part2_v6 (Autodesk Fusion 360 design; units mm, degrees)
Autodesk Fusion 360 part; units mm, degrees
sketch "Sketch1" plane through (0, 0, 0) normal (0, 1, 0) x (1, 0, 0)
  line L0 (5.0799, 0.3129) -> (55.0799, 0.3129)
  line L1 (55.0799, 0.3129) -> (55.0799, -174.6871)
  line L2 (55.0799, -174.6871) -> (5.0799, -174.6871)
  line L3 (5.0799, -174.6871) -> (5.0799, 0.3129)
  line L4 (30.0799, 0.3129) -> (30.0799, -174.6871) construction
  line L5 (5.0799, -94.6871) -> (55.0799, -94.6871)
  line L6 (55.0799, -94.6871) -> (55.0799, -79.6871)
  line L7 (55.0799, -79.6871) -> (5.0799, -79.6871)
  line L8 (5.0799, -79.6871) -> (5.0799, -94.6871)
  line L9 (5.0799, -94.6871) -> (55.0799, -79.6871) construction
  line L10 (55.0799, -94.6871) -> (5.0799, -79.6871) construction
  point P0 (30.0799, -87.1871)
  dimension "d2" = 175
  dimension "d11" = 50
  dimension "d12" = 15
  dimension "d37" = 50
  constraint horizontal L0
  constraint vertical L1
  constraint horizontal L2
  constraint midpoint L0 L4.start
  constraint midpoint L2 L4.end
  constraint horizontal L5
  constraint perpendicular L5 L6
  constraint parallel L5 L7
  constraint parallel L6 L8
  constraint coincident L9 P0
  constraint coincident L10 P0
  constraint midpoint L4 P0
  constraint vertical L3
  measures "d2" distance of L0.start L2.end
  measures "d11" distance of L6.end L7.end
  measures "d12" distance of L5.end L6.end
  measures "d37" distance of L0.start L0.end
extrude "Extrude1" add sketch "Sketch1" against normal blind 5
extrude "Extrude3" add sketch "Sketch1" along normal blind 45 contours L1 L3 L5 L6 L7 L8
sketch "Sketch2" plane through (0, 0, 94.6871) normal (0, 0, 1) x (1, 0, 0)
  line L0 (5.0799, 0) -> (55.0799, 0)
  line L1 (55.0799, 0) -> (55.0799, 45)
  line L2 (55.0799, 45) -> (5.0799, 45)
  line L3 (5.0799, 45) -> (5.0799, 0)
  circle A0 centre (30, 27.5) radius 5.35
  line L4 (55.0799, -5) -> (5.0799, -5)
  circle A1 centre (30, 27.5) radius 8
  line L5 (38, 27.5) -> (22, 27.5) construction
  line L6 (30, 19.5) -> (30, 35.5) construction
  circle A2 centre (22, 27.5) radius 2.05
  circle A3 centre (30, 19.5) radius 2.05
  circle A4 centre (38, 27.5) radius 2.05
  circle A5 centre (30, 35.5) radius 2.05
  circle A6 centre (30, 27.5) radius 11.5
  dimension "d15" = 10.7
  dimension "d16" = 32.5
  dimension "d17" = 16
  dimension "d18" = 4.1
  dimension "d19" = 4.1
  dimension "d20" = 4.1
  dimension "d21" = 4.1
  dimension "d24" = 23
  constraint concentric A0 A1
  constraint coincident A1 L5.start
  constraint coincident A1 L5.end
  constraint horizontal L5
  constraint coincident A1 L6.start
  constraint coincident A1 L6.end
  constraint perpendicular L5 L6
  constraint coincident L5.end A2.centre
  constraint coincident L6.start A3.centre
  constraint coincident L5.start A4.centre
  constraint coincident L6.end A5.centre
  constraint concentric A0 A6
  measures "d15" diameter of A0
  measures "d16" distance of A0.centre L4
  measures "d17" diameter of A1
  measures "d18" diameter of A2
  measures "d19" diameter of A3
  measures "d20" diameter of A4
  measures "d21" diameter of A5
  measures "d24" diameter of A6
extrude "Extrude4" cut sketch "Sketch2" against normal blind 24 contours A0 | A1 A4 | A1 A4 | A1 A5 | A1 A5 | A1 A3 | A1 A3 | A1 A2 | A1 A2
extrude "Extrude5" cut sketch "Sketch2" against normal blind 4 contours A0 | A1 A4 | A1 A4 | A1 A2 A3 A4 A5 | A1 A5 | A1 A5 | A1 A3 | A1 A3 | A1 A2 | A1 A2 | A6
extrude "Extrude6" cut sketch "Sketch2" along normal blind 5 from surface at -15 contours A0 | A1 A4 | A1 A4 | A1 A2 A3 A4 A5 | A1 A5 | A1 A5 | A1 A3 | A1 A3 | A1 A2 | A1 A2 | A6
sketch "Sketch3" plane through (0, 0, 0) normal (0, 1, 0) x (-1, 0, 0)
  line L0 (-5.0799, 79.6871) -> (-55.0799, 79.6871)
  line L1 (-5.0799, 94.6871) -> (-5.0799, 174.6871)
  line L2 (-55.0799, 174.6871) -> (-55.0799, 94.6871)
  line L3 (-55.0799, -0.3129) -> (-5.0799, -0.3129)
  line L4 (-55.0799, 94.6871) -> (-5.0799, 94.6871)
  line L5 (-5.0799, 174.6871) -> (-55.0799, 174.6871)
  line L6 (-55.0799, 79.6871) -> (-55.0799, -0.3129)
  line L7 (-5.0799, -0.3129) -> (-5.0799, 79.6871)
sketch "Sketch4" plane through (0, -5, 0) normal (0, -1, 0) x (1, 0, 0)
  line L0 (55.0799, 174.6871) -> (5.0799, 174.6871)
  line L1 (5.0799, 174.6871) -> (5.0799, -0.3129)
  line L2 (5.0799, -0.3129) -> (55.0799, -0.3129)
  line L3 (55.0799, -0.3129) -> (55.0799, 174.6871)
  line L4 (55.0799, -0.3129) -> (30.0799, -0.3129)
  line L5 (30.0799, -0.3129) -> (30.0799, 4.6871)
  line L6 (30.0799, 4.6871) -> (55.0799, 4.6871)
  line L7 (55.0799, 4.6871) -> (55.0799, -0.3129)
  line L8 (5.0799, 174.6871) -> (30.0799, 174.6871)
  line L9 (30.0799, 174.6871) -> (30.0799, 169.6871)
  line L10 (30.0799, 169.6871) -> (5.0799, 169.6871)
  line L11 (5.0799, 169.6871) -> (5.0799, 174.6871)
  line L12 (30.0799, -0.3129) -> (5.0799, -0.3129)
  line L13 (5.0799, -0.3129) -> (5.0799, 4.6871)
  line L14 (5.0799, 4.6871) -> (30.0799, 4.6871)
  line L15 (30.0799, 4.6871) -> (30.0799, -0.3129)
  line L16 (55.0799, 174.6871) -> (30.0799, 174.6871)
  line L17 (30.0799, 174.6871) -> (30.0799, 169.6871)
  line L18 (30.0799, 169.6871) -> (55.0799, 169.6871)
  line L19 (55.0799, 169.6871) -> (55.0799, 174.6871)
  circle A0 centre (20.0799, 157.1871) radius 2.5
  circle A1 centre (40.0799, 157.1871) radius 2.5
  circle A2 centre (20.0799, 17.1871) radius 2.5
  circle A3 centre (40.0799, 17.1871) radius 2.5
  dimension "d38" = 25
  dimension "d39" = 5
  dimension "d40" = 25
  dimension "d41" = 5
  dimension "d42" = 25
  dimension "d43" = 5
  dimension "d44" = 5
  dimension "d45" = 5
  dimension "d46" = 12.5
  dimension "d47" = 12.5
  dimension "d48" = 15
  dimension "d49" = 15
  dimension "d50" = 5
  dimension "d51" = 5
  dimension "d52" = 12.5
  dimension "d53" = 12.5
  dimension "d54" = 15
  dimension "d55" = 15
  constraint horizontal L4
  constraint vertical L5
  constraint horizontal L6
  constraint vertical L7
  constraint coincident L2.end L3.start
  constraint horizontal L8
  constraint vertical L9
  constraint horizontal L10
  constraint vertical L11
  constraint coincident L0.end L1.start
  constraint horizontal L12
  constraint vertical L13
  constraint horizontal L14
  constraint vertical L15
  constraint horizontal L16
  constraint vertical L17
  constraint horizontal L18
  constraint vertical L19
  constraint coincident L0.start L3.end
  measures "d38" distance of L5.end L6.end
  measures "d39" distance of L2.end L6.end
  measures "d40" distance of L0.end L8.end
  measures "d41" distance of L0.end L10.end
  measures "d42" distance of L4.end L1.end
  measures "d43" distance of L4.end L5.end
  measures "d44" diameter of A0
  measures "d45" diameter of A1
  measures "d46" distance of L10 A0.centre
  measures "d47" distance of L18 A1.centre
  measures "d48" distance of L3 A1.centre
  measures "d49" distance of L1 A0.centre
  measures "d50" diameter of A2
  measures "d51" diameter of A3
  measures "d52" distance of L6 A3.centre
  measures "d53" distance of L14 A2.centre
  measures "d54" distance of L1 A2.centre
  measures "d55" distance of L3 A3.centre
extrude "Extrude8" cut sketch "Sketch4" against normal blind 40 contours L0 L3 L9 L16 L17 L18 L19 | L1 L2 L5 L12 L13 L14 L15
extrude "Extrude9" add sketch "Sketch4" along normal blind 20 contours L0 L3 L9 L16 L17 L18 L19 | L0 L1 L8 L9 L10 L11 L17 | L2 L3 L4 L5 L6 L7 L15 | L1 L2 L5 L12 L13 L14 L15
extrude "Extrude10" cut sketch "Sketch4" against normal blind 35 contours A0 | A1 | A2 | A3
sketch "Sketch5" plane through (0, 0, 174.6871) normal (0, 0, 1) x (1, 0, 0)
  line L0 (30.0799, -5) -> (30.0799, 0)
  line L1 (30.0799, 0) -> (5.0799, 0)
  line L2 (5.0799, 0) -> (5.0799, -25)
  line L3 (5.0799, -25) -> (55.0799, -25)
  circle A0 centre (30.0799, -15) radius 2.5
  circle A1 centre (42.5799, -15) radius 2.5
  line L4 (55.0799, -25) -> (55.0799, -5)
  line L5 (55.0799, -5) -> (30.0799, -5)
  dimension "d62" = 5
  dimension "d63" = 10
  dimension "d64" = 5
  dimension "d69" = 25
  measures "d62" diameter of A0
  measures "d63" distance of L3 A0.centre
  measures "d64" diameter of A1
  measures "d69" distance of L2 A0.centre
extrude "Extrude12" add 2 faces at (13.4132, -5, 3.0204) (46.7466, -5, 171.3538) along direction (0, 1, 0) blind 5
extrude "Extrude13" cut sketch "Sketch5" against normal blind 200 contours A0
